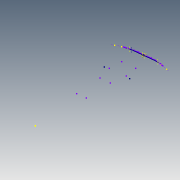
# Autodesk Inventor part: 6084-000 Lattice OSC, cesr
Saved by Autodesk Inventor 2020 (Build 240168000, 168)
## iProperties
RuleStatus: InUse
Shininess: 64.0
Length Units: 11269
Angle Units: 11279
Time Units: 11290
Mass Units: 11283
Length Display Precision: 3
Angle Display Precision: 2
Compacted: True
Part Number: 6084-000 Lattice OSC, cesr
Document SubType Name: Modeling
Created: 2002-07-16
Density: 1 g/cm^3
Material: Generic
Appearance: Default
Density: 0.0
Volumn: 0.0
Area: 0.0
PropertySet Name: Model Information
Control State: 0
Master: False
Checked Out: False
Autodesk Inventor part; units mm, degrees
ref_plane "Floor" through (0, 0, -1384.3) normal (0, 0, 1) x (1, 0, 0)
sketch "particles" plane through (0, 0, 0) normal (0, 0, 1) x (1, 0, 0)
  arc A0 (-19524.2026, 243365.6807) -> (-22776.2272, 242937.5935) centre (-9680.7789, 156022.4486) ccw
  arc A1 (-13807.3819, 243864.0227) -> (-16978.0813, 243652.624) centre (-13078.9412, 209054.5507) ccw
  arc A2 (11921.2114, 243903.412) -> (8969.1508, 243934.4) centre (8969.1508, 103305.42) ccw
  line L0 (-24861.8891, 242623.3482) -> (-22776.2272, 242937.5935)
  line L1 (-19524.2026, 243365.6807) -> (-16978.0813, 243652.624)
  arc A3 (16976.4822, 243652.7081) -> (13811.1004, 243863.731) centre (13080.2257, 209054.3101) ccw
  arc A4 (22786.6231, 242936.1085) -> (19515.9616, 243366.7278) centre (9679.8175, 156022.6756) ccw
  line L2 (16976.4822, 243652.7081) -> (19515.9616, 243366.7278)
  line L3 (15393.79, 243758.2) -> (15396.196, 243794.2906) construction
  line L4 (-15392.73, 243758.3) -> (-15395.1446, 243794.5157) construction
  line L5 (-21152.212, 243166.8082) -> (-21150.21, 243151.6) construction
  arc A5 (-8973.0365, 243934.4) -> (-11915.2657, 243903.6181) centre (-8973.0365, 103305.42) ccw
  line L6 (-11915.2657, 243903.6181) -> (-13807.3819, 243864.0227)
  line L7 (-8973.0365, 243934.4) -> (8969.1508, 243934.4)
  line L8 (22786.6231, 242936.1085) -> (24870.238, 242621.8932)
  line L9 (11921.2114, 243903.412) -> (13811.1004, 243863.731)
  line L10 (10445.2624, 243926.6528) -> (10445.18, 243918.8) construction
  line L11 (-10444.2316, 243926.7043) -> (-10444.15, 243918.9) construction
  line L12 (21153.3128, 243166.7637) -> (21151.29, 243151.4) construction
  line L13 (31299.4576, 241280.1593) -> (35040.3137, 240277.7766)
  arc A6 (31299.4576, 241280.1593) -> (24870.238, 242621.8932) centre (16131.5115, 184673.9281) ccw
  arc A7 (-24861.8891, 242623.3482) -> (-31301.0844, 241279.8288) centre (-16130.7349, 184674.2417) ccw
  line L14 (-39021.3143, 239211.1683) -> (-35039.2345, 240278.1795) construction
  line L15 (-28081.51, 241951.7) -> (-28100.3519, 242042.005) construction
  line L16 (28082.61, 241951.4) -> (28101.4362, 242041.6272) construction
  arc A8 (-39021.3143, 239211.1683) -> (-45263.6703, 237157.0456) centre (-23853.4838, 182604.9061) ccw construction
  line L17 (-42142.49, 238184.1) -> (-42171.3081, 238271.6764) construction
  line L18 (-45263.6703, 237157.0456) -> (-53973.0439, 233738.8604) construction
  arc A9 (45264.6776, 237156.6444) -> (39022.3653, 239210.7644) centre (23854.4192, 182604.5331) ccw construction
  line L19 (42172.337, 238271.2727) -> (42143.52, 238183.7) construction
  line L20 (45264.6776, 237156.6444) -> (53861.2746, 233782.7078) construction
  line L21 (-35039.24, 240278.2) -> (-35039.2345, 240278.1795) construction
  line L22 (-35039.2345, 240278.1795) -> (-35039.1899, 240278.0131) construction
  line L23 (-35039.2345, 240278.1795) -> (-31301.0844, 241279.8288)
  line L24 (35040.32, 240277.8) -> (35040.3137, 240277.7766) construction
  line L25 (35040.3137, 240277.7766) -> (39022.3653, 239210.7644) construction
  line L26 (-27217.9131, 242219.0632) -> (-27162.1286, 241951.7) construction
  point P0 (0, 0)
  point P1 (-24387.66, 242694.8)
  point P2 (-18831.03, 243443.8)
  point P3 (-12542.13, 243890.5)
  point P4 (-5285.354, 243934.4)
  point P5 (-241.1875, 243934.3)
  point P6 (233.8125, 243934.3)
  point P7 (-2.2572, 243934.3)
  point P8 (5300.592, 243934.3)
  point P9 (13007.68, 243880.6)
  point P10 (18375.14, 243495.2)
  point P11 (24388.77, 242694.5)
  point P12 (32432.33, 240976.6)
  point P13 (-32431.24, 240977)
  point P14 (-32431.24, 240977)
  point P15 (-24387.66, 242694.8)
  point P16 (-18831.03, 243443.8)
  point P17 (-12542.13, 243890.5)
  point P18 (-28540.5126, 241948.4018)
  point P19 (38556.11, 239335.7)
  point P20 (36139.07, 239983.4)
  point P21 (33941.58, 240572.2)
  point P22 (-33940.51, 240572.6)
  point P23 (-36137.98, 239983.7)
  point P24 (-38555.07, 239336.1)
  point P25 (48937.65, 235715.1)
  point P26 (-48936.66, 235715.5)
  dimension "B46W_y" = 241951.7
  dimension "Q46W_z" = 0
  dimension "d473" = 3280.0797
  dimension "d474" = 3288.9315
  dimension "d475" = 2952.2233
  dimension "d476" = 3172.408
  dimension "d477" = 3298.8876
  dimension "d482" = 2942.3902
  dimension "d513" = 34817.093
  dimension "d514" = 87896.15
  dimension "d515" = 140628.98
  dimension "d516" = 140628.98
  dimension "d517" = 34817.093
  dimension "d518" = 87896.15
  dimension "d523" = 58603.174
  dimension "d529" = 58603.174
  dimension "d535" = 92.2497
  dimension "d538" = 3288.9315
  dimension "d539" = 92.1704
  dimension "d635" = 58603.174
  dimension "d664" = 0.1935
  dimension "d669" = 900
  dimension "d671" = 450
  constraints: 54 end point, 32 point on circle, 22 tangent, 15 point on line, 10 centre point, 10 line through centre, 6 perpendicular, 5 coincident, 1 equal radius, 1 horizontal, 1 horizontal alignment, 1 parallel
  measures "d473" distance of L1.start L0.end
  measures "d474" distance of L15.start L0.start
  measures "d475" distance of L9.start L7.end
  measures "d476" distance of L2.start L9.end
  measures "d477" distance of L8.start L2.end
  measures "d482" distance of L7.start L6.start
  measures "d513" radius of A1
  measures "d514" radius of A0
  measures "d515" radius of A5
  measures "d516" radius of A2
  measures "d517" radius of A3
  measures "d518" radius of A4
  measures "d523" radius of A6
  measures "d529" radius of A7
  measures "d535" distance of L15.start L15.end
  measures "d538" distance from line of L23.end L15
  measures "d539" distance of L16.start L16.end
  measures "d635" radius of A8
  measures "d664" distance of L21.start L22.end
  measures "d669" distance between parallel lines of L15 L26
  measures "d671" distance from line of point (-28540.513, 241948.402) L15
sketch "Detector Steel Sketch" plane through (0, 0, 0) normal (0, 0, 1) x (1, 0, 0)
  line L0 (-1712.2572, 242017.1771) -> (1707.7428, 242017.1771)
  line L1 (1707.7428, 242017.1771) -> (1707.7428, 241305.1771)
  line L2 (1707.7428, 241305.1771) -> (-1712.2572, 241305.1771)
  line L3 (-1712.2572, 241305.1771) -> (-1712.2572, 242017.1771)
  line L4 (-2.2572, 243934.3) -> (-2.2572, 243272.085) construction
  point P0 (0, 0)
  point P1 (-1712.2572, 242118.2)
  point P2 (1707.7428, 242118.2)
  dimension "d550" = 1917.1229
  dimension "d569" = 3420
  dimension "d570" = 712
  dimension "d586" = 1816.1
  dimension "d587" = 101.0229
  constraints: 10 end point, 2 parallel, 2 point on line, 1 horizontal, 1 horizontal alignment, 1 perpendicular, 1 symmetric about line, 1 vertical
  measures "d550" distance from line of L0 L4.start
  measures "d569" distance of L1.end L2.end
  measures "d570" distance of L0.end L1.end
  measures "d586" vertical distance of L4.start point (-1712.257, 242118.2)
  measures "d587" distance from line of L0 point (-1712.257, 242118.2)
extrude "Detector Steel" add sketch "Detector Steel Sketch" along normal blind 532.75
sketch "extraction path" plane through (0, 0, 0) normal (0, 0, 1) x (1, 0, 0)
  line L0 (-28555.0758, 242015.6147) -> (-25555.0758, 242015.6147)
  line L1 (-28081.51, 241951.7) -> (-28100.3519, 242042.005) construction
  line L2 (28082.61, 241951.4) -> (28101.4362, 242041.6272) construction
  line L3 (28554.696, 242015.6147) -> (25554.696, 242015.6147)
  line L4 (-35039.24, 240278.2) -> (-28555.0758, 242015.6147)
  line L5 (-28540.5126, 241948.4018) -> (-28548.2297, 241984.0185) construction
  arc A0 (-24861.8891, 242623.3482) -> (-31301.0844, 241279.8288) centre (-16130.7349, 184674.2417) ccw construction
  arc A1 (31299.4576, 241280.1593) -> (24870.238, 242621.8932) centre (16131.5115, 184673.9281) ccw construction
  line L6 (28554.696, 242015.6147) -> (35040.32, 240277.8)
  line L7 (-25555.0758, 242015.6147) -> (-1712.2572, 242118.2) construction
  line L8 (1707.7428, 242118.2) -> (25554.696, 242015.6147) construction
  line L9 (-28645.0743, 242003.7661) -> (-28462.5976, 242027.7897) construction
  line L10 (-28645.0743, 242003.7661) -> (-35039.24, 240278.2) construction
  line L11 (-35039.24, 240278.2) -> (-28462.5976, 242027.7897) construction
  line L12 (-28555.0758, 242015.6147) -> (-28574.0241, 242159.5416) construction
  line L13 (-25555.0758, 242015.6147) -> (-25555.0758, 242044.1016) construction
  line L14 (-28645.0743, 242003.7661) -> (-25555.0758, 241998.2381) construction
  line L15 (-28462.5976, 242027.7897) -> (-25555.0758, 242032.9912) construction
  point P0 (0, 0)
  dimension "B46W_y" = 241951.7
  dimension "d544" = 3000
  dimension "d566" = 3000
  dimension "d567" = 68.7725
  dimension "d580" = 6714.4113
  dimension "d581" = 6712.8977
  dimension "d639" = 0.205
  dimension "d640" = 0.103
  dimension "d641" = 184.0514
  dimension "d642" = 23.6967
  dimension "d643" = 7.5
  dimension "d656" = 0.247
  dimension "d665" = 0.205
  dimension "d666" = 0.103
  dimension "d667" = 34.7531
  constraints: 28 end point, 4 coincident, 2 horizontal, 2 perpendicular, 2 point on line, 2 tangent, 2 vertical alignment, 1 horizontal alignment, 1 line through centre
  measures "d544" distance of L0.start L0.end
  measures "d566" distance of L3.start L3.end
  measures "d567" distance of L5.start L0.start
  measures "d580" distance of L6.end L3.start
  measures "d581" distance of L4.start L0.start
  measures "d639" angle of L11 L10
  measures "d640" angle of L10 L4
  measures "d641" distance of L9.start L9.end
  measures "d642" distance from line of L11 L9.start
  measures "d643" angle of L9 L0
  measures "d656" angle of L0 L7
  measures "d665" angle of L14 L15
  measures "d666" angle of L14 L0
  measures "d667" distance of L14.end L15.end
ref_plane "West Path Plane" through (-25555.0758, 242015.6147, 0) normal (0.0043, -1, 0) x (1, 0.0043, 0)
ref_plane "East Path Plane" through (1707.7428, 242118.2, 0) normal (-0.0043, -1, 0) x (1, -0.0043, 0)
sketch "West Path" plane through (-25555.0758, 242015.6147, 0) normal (0.0043, -1, 0) x (1, 0.0043, 0)
  line L0 (0, 0) -> (3979.9497, 400)
  line L1 (3979.9497, 400) -> (23843.0392, 400)
  line L2 (3979.9497, 400) -> (3978.4479, 429.9609) construction
  line L3 (3978.4479, 429.9609) -> (3955.0751, 397.5) construction
  line L4 (3978.4479, 429.9609) -> (4004.9497, 400) construction
  line L5 (3979.9497, 400) -> (4003.8883, 401.1999) construction
  point P0 (24513.5604, 0)
  point P1 (0, 0)
  point P2 (23843.0392, 0)
  dimension "d574" = 5.739
  dimension "d576" = 400
  dimension "d582" = 4000
  dimension "d583" = 19863.0895
  dimension "d678" = 25
  dimension "d679" = 25
  dimension "d683" = 40
  constraints: 12 end point, 3 point on line, 1 coincident, 1 equal length, 1 horizontal, 1 perpendicular, 1 vertical alignment
  measures "d574" angle of L0 L1
  measures "d576" distance from line of L1 L0.start
  measures "d582" distance of L0.start L0.end
  measures "d583" distance of L0.end L1.end
  measures "d678" distance of L3.end L0.end
  measures "d679" distance of L4.end L0.end
  measures "d683" distance of L2.end L3.end
sketch "East Path" plane through (1707.7428, 242118.2, 0) normal (-0.0043, -1, 0) x (1, -0.0043, 0)
  line L0 (23847.1738, 0) -> (19867.2241, 400)
  line L1 (19867.2241, 400) -> (0, 400)
  line L2 (19867.2241, 400) -> (19869.0357, 436.1406) construction
  line L3 (19869.0357, 436.1406) -> (19892.0988, 397.5) construction
  line L4 (19842.2241, 400) -> (19869.0357, 436.1406) construction
  line L5 (19867.2241, 400) -> (19891.3278, 398.7918) construction
  point P0 (0, 0)
  point P1 (-3419.9684, 400)
  dimension "d577" = 5.739
  dimension "d578" = 4000
  dimension "d579" = 19867.2241
  dimension "d684" = 25
  dimension "d685" = 25
  dimension "d686" = 45
  constraints: 12 end point, 3 point on line, 1 equal length, 1 horizontal, 1 horizontal alignment, 1 perpendicular, 1 vertical alignment
  measures "d577" angle of L1 L0
  measures "d578" distance of L0.start L0.end
  measures "d579" distance of L0.end L1.end
  measures "d684" distance of L4.start L0.end
  measures "d685" distance of L3.end L0.end
  measures "d686" distance of L4.start L2.end
ref_plane "Amplifier Plane" through (-1712.2572, 242118.2, 400) normal (0, 0, 1) x (1, 0, 0)
sketch "Amplifier Sketch" plane through (-1712.2572, 242118.2, 400) normal (0, 0, 1) x (1, 0, 0)
  line L0 (0, 0) -> (3420, 0)
  line L1 (1196.5296, -13.4704) -> (1223.4704, 13.4704) construction
  line L2 (1210, 0) -> (1210, 100) construction
  line L3 (1223.4704, 113.4704) -> (1196.5296, 86.5296) construction
  line L4 (1210, 100) -> (2210, 100) construction
  line L5 (2196.5296, 113.4704) -> (2223.4704, 86.5296) construction
  line L6 (2196.5296, 13.4704) -> (2223.4704, -13.4704) construction
  line L7 (2210, 100) -> (2210, 0) construction
  point P0 (1712.2572, -242118.2)
  point P1 (1710, 100)
  point P2 (1710, 0)
  dimension "d584" = 3420
  dimension "d674" = 45
  dimension "d675" = 100
  dimension "d676" = 38.1
  dimension "d677" = 1000
  constraints: 16 end point, 6 midpoint, 3 equal length, 2 horizontal, 2 parallel, 2 point on line, 2 vertical alignment, 1 perpendicular, 1 vertical
  measures "d584" distance of L0.start L0.end
  measures "d674" angle of L1 L0
  measures "d675" distance of L2.start L2.end
  measures "d676" distance of L1.start L1.end
  measures "d677" distance of L2.end L4.end
sketch "total path length curve" plane through (0, 0, 0) normal (0, 0, 1) x (1, 0, 0)
  line L0 (-35291.0685, 241267.4477) -> (35286.554, 241267.4477)
  point P0 (0, 0)
  point P1 (-2.2572, 243934.3)
  point P2 (-2.2572, 241267.4477)
  dimension "d585" = 70577.6226
  constraints: 2 end point, 1 horizontal, 1 midpoint, 1 vertical alignment
  measures "d585" distance of L0.start L0.end
ref_plane "M46E02 sketch plane" through (25554.696, 242015.6147, 0) normal (0, -0.9991, 0.0428) x (-0.995, 0.0043, 0.1)
sketch "M46E02 sketch" plane through (25554.696, 242015.6147, 0) normal (0, -0.9991, 0.0428) x (-0.995, 0.0043, 0.1)
  line L0 (0, 0) -> (1.6287, -32.462) construction
  line L1 (0, 0) -> (4000, 0) construction
  line L2 (-2984.9347, -300.2747) -> (0, 0) construction
  line L3 (1.6287, -32.462) -> (25, 0) construction
  line L4 (1.6287, -32.462) -> (-24.8745, -2.5023) construction
  line L5 (0, 0) -> (-32.462, -1.6287) construction
  point P0 (24390.4864, 12855.1593)
  dimension "d693" = 25
  dimension "d694" = 25
  dimension "d695" = 40
  constraints: 8 end point, 2 equal length, 2 point on line, 1 perpendicular
  measures "d693" distance of L0.start L3.end
  measures "d694" distance of L0.start L4.end
  measures "d695" distance of L0.end L3.end
ref_plane "M46W02 sketch plane" through (-28555.0758, 242015.6147, 0) normal (0, -0.9991, 0.0428) x (1, 0, 0)
sketch "M46W02 sketch" plane through (-28555.0758, 242015.6147, 0) normal (0, -0.9991, 0.0428) x (1, 0, 0)
  line L0 (0, 0) -> (3000, 0) construction
  line L1 (3000, 0) -> (6979.9129, 400.3664) construction
  line L2 (3000, 0) -> (2998.0613, 38.6417) construction
  line L3 (2998.0613, 38.6417) -> (2975, 0) construction
  line L4 (2998.0613, 38.6417) -> (3024.8745, 2.5023) construction
  line L5 (3000, 0) -> (3038.6417, 1.9387) construction
  point P0 (28555.0758, -10351.1132)
  dimension "d702" = 25
  dimension "d703" = 25
  dimension "d704" = 45
  constraints: 8 end point, 2 equal length, 2 point on line, 1 perpendicular
  measures "d702" distance of L3.end L0.end
  measures "d703" distance of L4.end L0.end
  measures "d704" distance of L2.end L3.end
equation "\"B46W_y\" = 241951.7"
equation "\"Q46W_z\" = 0"
equation "\"IPx\" = 0"
equation "\"IPy\" = 0"
equation "\"IPz\" = 0"
equation "\"IPax\" = 0"
equation "\"IPay\" = 0"
equation "\"IPaz\" = 0"
equation "\"OSC_PICKUP_1_x\" = -36137.98"
equation "\"OSC_PICKUP_1_y\" = 239983.7"
equation "\"OSC_PICKUP_1_z\" = 0"
equation "\"OSC_PICKUP_1_ax\" = 0"
equation "\"OSC_PICKUP_1_ay\" = 0"
equation "\"OSC_PICKUP_1_az\" = 344.999698deg"
equation "\"P_MARK_x\" = -35039.24"
equation "\"P_MARK_y\" = 240278.2"
equation "\"P_MARK_z\" = 0"
equation "\"P_MARK_ax\" = 0"
equation "\"P_MARK_ay\" = 0"
equation "\"P_MARK_az\" = 344.999698deg"
equation "\"OSC_START_x\" = -35039.24"
equation "\"OSC_START_y\" = 240278.2"
equation "\"OSC_START_z\" = 0"
equation "\"OSC_START_ax\" = 0"
equation "\"OSC_START_ay\" = 0"
equation "\"OSC_START_az\" = 344.999698deg"
equation "\"OSC_PICKUP_2_x\" = -33940.51"
equation "\"OSC_PICKUP_2_y\" = 240572.6"
equation "\"OSC_PICKUP_2_z\" = 0"
equation "\"OSC_PICKUP_2_ax\" = 0"
equation "\"OSC_PICKUP_2_ay\" = 0"
equation "\"OSC_PICKUP_2_az\" = 344.999698deg"
equation "\"DET_45W_x\" = -32779.36"
equation "\"DET_45W_y\" = 240883.7"
equation "\"DET_45W_z\" = 0"
equation "\"DET_45W_ax\" = 0"
equation "\"DET_45W_ay\" = 0"
equation "\"DET_45W_az\" = 344.999698deg"
equation "\"Q45W_x\" = -32431.24"
equation "\"Q45W_y\" = 240977"
equation "\"Q45W_z\" = 0"
equation "\"Q45W_ax\" = 0"
equation "\"Q45W_ay\" = 0"
equation "\"Q45W_az\" = 344.999698deg"
equation "\"SEX_45W_x\" = -31947.79"
equation "\"SEX_45W_y\" = 241106.4"
equation "\"SEX_45W_z\" = 0"
equation "\"SEX_45W_ax\" = 0"
equation "\"SEX_45W_ay\" = 0"
equation "\"SEX_45W_az\" = 344.999698deg"
equation "\"B46W_x\" = -28081.51"
equation "\"B46W_z\" = 0"
equation "\"B46W_ax\" = 0"
equation "\"B46W_ay\" = 0"
equation "\"B46W_az\" = 348.213992deg"
equation "\"Q46W_x\" = -24387.66"
equation "\"Q46W_y\" = 242694.8"
equation "\"Q46W_ax\" = 0"
equation "\"Q46W_ay\" = 0"
equation "\"Q46W_az\" = 351.428285deg"
equation "\"DET_46W_x\" = -24014.47"
equation "\"DET_46W_y\" = 242751"
equation "\"DET_46W_z\" = 0"
equation "\"DET_46W_ax\" = 0"
equation "\"DET_46W_ay\" = 0"
equation "\"DET_46W_az\" = 351.428285deg"
equation "\"B47W_x\" = -21150.21"
equation "\"B47W_y\" = 243151.6"
equation "\"B47W_z\" = 0"
equation "\"B47W_ax\" = 0"
equation "\"B47W_ay\" = 0"
equation "\"B47W_az\" = 352.499773deg"
equation "\"DET_47W_x\" = -19175.25"
equation "\"DET_47W_y\" = 243405"
equation "\"DET_47W_z\" = 0"
equation "\"DET_47W_ax\" = 0"
equation "\"DET_47W_ay\" = 0"
equation "\"DET_47W_az\" = 353.571204deg"
equation "\"Q47W_x\" = -18831.03"
equation "\"Q47W_y\" = 243443.8"
equation "\"Q47W_z\" = 0"
equation "\"Q47W_ax\" = 0"
equation "\"Q47W_ay\" = 0"
equation "\"Q47W_az\" = 353.571204deg"
equation "\"SEX_47W_x\" = -18316.39"
equation "\"SEX_47W_y\" = 243501.8"
equation "\"SEX_47W_z\" = 0"
equation "\"SEX_47W_ax\" = 0"
equation "\"SEX_47W_ay\" = 0"
equation "\"SEX_47W_az\" = 353.571204deg"
equation "\"B47AW_x\" = -15392.73"
equation "\"B47AW_y\" = 243758.3"
equation "\"B47AW_z\" = 0"
equation "\"B47AW_ax\" = 0"
equation "\"B47AW_ay\" = 0"
equation "\"B47AW_az\" = 356.185439deg"
equation "\"DET_I47AW_x\" = -13007.03"
equation "\"DET_I47AW_y\" = 243880.8"
equation "\"DET_I47AW_z\" = 0"
equation "\"DET_I47AW_ax\" = 0"
equation "\"DET_I47AW_ay\" = 0"
equation "\"DET_I47AW_az\" = 358.799731deg"
equation "\"Q47AW_x\" = -12542.13"
equation "\"Q47AW_y\" = 243890.5"
equation "\"Q47AW_z\" = 0"
equation "\"Q47AW_ax\" = 0"
equation "\"Q47AW_ay\" = 0"
equation "\"Q47AW_az\" = 358.799731deg"
equation "\"B48W_x\" = -10444.15"
equation "\"B48W_y\" = 243918.9"
equation "\"B48W_z\" = 0"
equation "\"B48W_ax\" = 0"
equation "\"B48W_ay\" = 0"
equation "\"B48W_az\" = 359.399732deg"
equation "\"DET_I48W_x\" = -8261.196"
body "Solid1"
